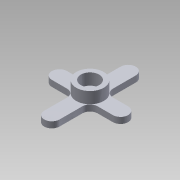
# Autodesk Inventor part: CoronaArm
Saved by Autodesk Inventor 2014 (Build 180170000, 170)
## iProperties
Created: 2013-11-13
Part Number: CoronaArm
Material: Générique
Document SubType Name: Modeling
Designer: Grégoire
Density: 1 g/cm^3
Appearance: Par défaut
Author: Grégoire
Autodesk Inventor part; units mm, degrees
ref_plane "YZ Plane" through (0, 0, 0) normal (1, 0, 0) x (0, 1, 0)
ref_plane "XZ Plane" through (0, 0, 0) normal (0, 1, 0) x (-1, 0, 0)
ref_plane "XY Plane" through (0, 0, 0) normal (0, 0, 1) x (1, 0, 0)
sketch "Esquisse1" plane through (0, 0, 0) normal (0, 0, 1) x (1, 0, 0)
  line L0 (-8.7953, 10.6752) -> (-4.7953, 10.6752)
  line L1 (-4.7953, -13.3248) -> (-8.7953, -13.3248)
  line L2 (3.2047, -3.3248) -> (3.2047, 0.6752)
  line L3 (-16.7953, 0.6752) -> (-16.7953, -3.3248)
  line L4 (3.2047, 0.6752) -> (-4.7953, 0.6752)
  line L5 (-8.7953, 0.6752) -> (-16.7953, 0.6752)
  line L6 (-4.7953, 10.6752) -> (-4.7953, 0.6752)
  line L7 (-4.7953, -3.3248) -> (-4.7953, -13.3248)
  line L8 (-16.7953, -3.3248) -> (-8.7953, -3.3248)
  line L9 (-4.7953, -3.3248) -> (3.2047, -3.3248)
  line L10 (-8.7953, -13.3248) -> (-8.7953, -3.3248)
  line L11 (-8.7953, 0.6752) -> (-8.7953, 10.6752)
  line L12 (-8.7953, 0.6752) -> (-4.7953, -3.3248) construction
  line L13 (-8.7953, -3.3248) -> (-4.7953, 0.6752) construction
  circle A0 centre (-6.7953, -1.3248) radius 1
  dimension "d0" = 10
  dimension "d1" = 8
  dimension "d2" = 4
  dimension "d5" = 2
  constraints: 28 end point, 10 parallel, 7 equal length, 5 perpendicular, 3 horizontal, 1 centre point, 1 midpoint
  measures "d0" distance of L0.end L4.end
  measures "d1" distance of L7.start L2.start
  measures "d2" distance of L0.start L0.end
  measures "d5" diameter of A0
extrude "Extrusion2" add sketch "Esquisse1" along normal blind 1.6
fillet "Congé1" radius 2 12 edges at (-8.7953, 0.6752, 0.8) (-8.7953, -3.3248, 0.8) (-16.7953, -3.3248, 0.8) (-16.7953, 0.6752, 0.8) (-8.7953, 10.6752, 0.8) (-4.7953, 10.6752, 0.8) (-4.7953, 0.6752, 0.8) (3.2047, 0.6752, 0.8) (3.2047, -3.3248, 0.8) (-4.7953, -3.3248, 0.8) (-4.7953, -13.3248, 0.8) (-8.7953, -13.3248, 0.8)
sketch "Esquisse2" plane through (0, 0, 1.6) normal (0, 0, 1) x (1, 0, 0)
  circle A0 centre (-6.7953, -1.3248) radius 1 construction
  circle A1 centre (-6.7953, -1.3248) radius 3.6
  circle A2 centre (-6.7953, -1.3248) radius 2.4
  point P0 (0, 0)
  dimension "d8" = 1.2
  dimension "d9" = 7.2
  constraints: 2 centre point, 2 coincident
  measures "d8" radial gap between concentric circles of A1 A2
  measures "d9" diameter of A1
extrude "Extrusion3" add sketch "Esquisse2" along normal blind 3
